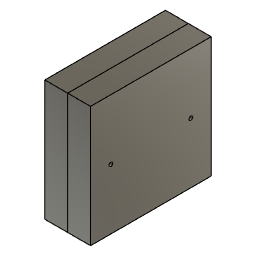
silicone_mold_tyres (Autodesk Fusion 360 design; units mm, degrees)
Autodesk Fusion 360 part; units mm, degrees
note: some values were not read from the file. Set by a fixed rule: which face or edge a step refers to.
sketch "Sketch1" plane through (0, 0, 0) normal (0, 0, 1) x (1, 0, 0)
  circle A0 centre (0, 0) radius 25
  dimension "d1" = 50
  constraint coincident A0.centre origin
  measures "d1" diameter of A0
extrude "Extrude1" add sketch "Sketch1" along normal blind 18 makes body 1
move_body "Move1" bodies 1 to x (0, 0, 1) y (0, 1, 0) z (-1, 0, 0) at (18, 0, 18)
fillet "Fillet1" radius 4 2 edges at (0, -9.0404, -5.3082) (18, -9.0404, -5.3082) on bodies 1
ref_plane "WorkPlane1" through (9, 0, 18) normal (1, 0, 0) x (0, 0, -1)
sketch "Sketch2" plane through (9, 0, 18) normal (1, 0, 0) x (0, 1, 0)
  line L0 (0, 0) -> (-26.2939, 0)
  circle A0 centre (0, 0) radius 26.2939
  circle A1 centre (0, 0) radius 25
  circle A2 centre (0, 0) radius 25
  constraint coincident L0.start A0.centre
  constraint horizontal L0
  constraint coincident L0.end A0
extrude "Extrude2" add sketch "Sketch2" along normal mid plane 9.2 separate body makes body 2
move_face "OffsetFaces1" offset -0.5 1 faces at (7.4667, -26.1632, 15.382) on bodies 2
sketch "Sketch3" plane through (0, 0, 0) normal (0, 1, 0) x (1, 0, 0)
  line L0 (-4.0723, -11.8438) -> (22.6184, -22.2298)
  line L1 (-4.767, -13.6293) -> (21.9237, -24.0153)
  line L2 (21.9237, -24.0153) -> (22.6184, -22.2298)
  line L3 (-4.767, -13.6293) -> (-4.0723, -11.8438)
  line L4 (4.4, 7.7939) -> (4.4, -43.7939)
  line L5 (13.6, -43.7939) -> (13.6, 7.7939)
  circle A0 through (4, 7, 0) (4, -30.5, 21.6506) (4, -30.5, -21.6506)
  line L6 (4, -18) -> (24.1536, -18)
  line L7 (-4.0723, -24.1562) -> (22.6184, -13.7702)
  line L8 (-4.767, -22.3707) -> (-4.0723, -24.1562)
  line L9 (-4.767, -22.3707) -> (21.9237, -11.9847)
  line L10 (21.9237, -11.9847) -> (22.6184, -13.7702)
  dimension "d9" = 1.9159
  constraint perpendicular L0 L2
  constraint perpendicular L0 L3
  constraint perpendicular L4 L6
  constraint symmetric L0.start L6 L7.start
  constraint symmetric L0.end L6 L7.end
  constraint symmetric L1.start L6 L8.start
  constraint symmetric L1.end L6 L9.end
extrude "Extrude3" cut sketch "Sketch3" against normal blind 58 contours L0 L1 L3 L4 | L0 L1 L4 L9 | L0 L6 L9 | L1 L6 L7 | L0 L1 L5 L7 | L0 L1 L2 L5 keep common part bodies 2
pattern_circular "C-Pattern1" count 23 over 360 about axis through (14, 0, 18) along (-1, 0, 0) of bodies 2 makes body 3 at (7.9822, -24.2718, 23.9901) makes body 4 at (7.9822, -21.7556, 30.3164) makes body 5 at (7.9822, -17.6259, 35.7293) makes body 6 at (7.9822, -12.189, 39.8272) makes body 7 at (7.9822, -5.8481, 42.3064) makes body 8 at (7.9822, 0.9265, 42.9828) makes body 9 at (7.9822, 7.6325, 41.8064) makes body 10 at (7.9822, 13.7723, 38.8644) makes body 11 at (7.9822, 18.8908, 34.375) makes body 12 at (7.9822, 22.6081, 28.6711) makes body 13 at (7.9822, 24.6488, 22.1757) makes body 14 at (7.9822, 24.8614, 15.3707) makes body 15 at (7.9822, 23.2301, 8.7607) makes body 16 at (7.9822, 19.8759, 2.8359) makes body 17 at (7.9822, 15.0476, -1.9642) makes body 18 at (7.9822, 9.1034, -5.2837) makes body 19 at (7.9822, 2.4839, -6.8763) makes body 20 at (7.9822, -4.3197, -6.624) makes body 21 at (7.9822, -10.803, -4.5454) makes body 22 at (7.9822, -16.4851, -0.7947) makes body 23 at (7.9822, -20.9445, 4.3499) makes body 24 at (7.9822, -23.8506, 10.5068)
sketch "Sketch4" plane through (0, 0, 0) normal (-1, 0, 0) x (0, -1, 0)
  circle A0 centre (0, 18) radius 21
  circle A1 centre (0, 18) radius 17.4465
  constraint concentric A0 A1
extrude "Extrude4" cut sketch "Sketch4" against normal blind 40 contours A1 bodies 1
sketch "Sketch5" plane through (0, 0, 0) normal (-1, 0, 0) x (0, -1, 0)
  circle A0 centre (0, 18) radius 17.4465
  circle A1 centre (0, 18) radius 21
  line L0 (29, 47) -> (-29, 47)
  line L1 (-29, 47) -> (-29, -11)
  line L2 (-29, -11) -> (29, -11)
  line L3 (29, -11) -> (29, 47)
  line L4 (29, 47) -> (-29, -11) construction
  line L5 (-29, 47) -> (29, -11) construction
  point P0 (0, 18)
  dimension "d16" = 58
  dimension "d17" = 58
  constraint horizontal L0
  constraint perpendicular L0 L1
  constraint parallel L0 L2
  constraint parallel L1 L3
  constraint coincident L4 P0
  constraint coincident L5 P0
  constraint coincident P0 A0.centre
  measures "d16" distance of L1.end L2.end
  measures "d17" distance of L0.end L1.end
extrude "Extrude5" add sketch "Sketch5" against normal blind 20 separate body contours A0 | A1 | L0 L1 L2 L3 makes body 25
extrude "Extrude6" add sketch "Sketch5" along normal blind 2 separate body contours A0 | A1 | L0 L1 L2 L3 makes body 26
combine "Combine1" operation add target body 25 tool bodies 26
combine "Combine2" operation add target body 1 tool bodies 2 9 18 10 11 17 3 7 24 14 12 13 15 16 6 21 4 5 22 23 8 20 19
combine "Combine3" operation add target body 25 tool bodies 1 keep tools
ref_plane "WorkPlane2" through (9, 0, 18) normal (1, 0, 0) x (0, 0, -1)
split "Split1" by plane through (9, 0, 18) normal (1, 0, 0) bodies 25 makes body 27 at (20, 9.6667, 27.6667)
combine "Combine4" operation cut target body 27 tool bodies 1 keep tools
combine "Combine5" operation cut target body 25 tool bodies 1 keep tools
sketch "Sketch6" plane through (9, 0, 0) normal (1, 0, 0) x (0, 1, 0)
  line L0 (-25.775, 18.9864) -> (-24.9805, 18.9864)
  arc A0 (-24.3394, 23.7089) -> (-24.9805, 18.9864) centre (0, 18) ccw
  line L1 (-24.3394, 23.7089) -> (-25.1046, 23.9233)
  arc A1 (-24.5531, 25.9038) -> (-25.1046, 23.9233) centre (0, 18) ccw
  line L2 (-24.5531, 25.9038) -> (-23.7881, 25.6895)
  arc A2 (-21.8966, 30.0639) -> (-23.7881, 25.6895) centre (0, 18) ccw
  line L3 (-21.8966, 30.0639) -> (-22.5755, 30.4768)
  arc A3 (-21.5102, 32.2351) -> (-22.5755, 30.4768) centre (0, 18) ccw
  line L4 (-21.5102, 32.2351) -> (-20.8313, 31.8223)
  arc A4 (-17.8298, 35.5242) -> (-20.8313, 31.8223) centre (0, 18) ccw
  line L5 (-17.8298, 35.5242) -> (-18.3722, 36.1049)
  arc A5 (-16.872, 37.5106) -> (-18.3722, 36.1049) centre (0, 18) ccw
  line L6 (-16.872, 37.5106) -> (-16.3297, 36.9299)
  arc A6 (-12.4407, 39.6848) -> (-16.3297, 36.9299) centre (0, 18) ccw
  line L7 (-12.4407, 39.6848) -> (-12.8062, 40.3903)
  arc A7 (-10.9824, 41.3391) -> (-12.8062, 40.3903) centre (0, 18) ccw
  line L8 (-10.9824, 41.3391) -> (-10.6169, 40.6336)
  arc A8 (-6.1288, 42.2371) -> (-10.6169, 40.6336) centre (0, 18) ccw
  line L9 (-6.1288, 42.2371) -> (-6.2905, 43.0151)
  arc A9 (-4.2783, 43.4366) -> (-6.2905, 43.0151) centre (0, 18) ccw
  line L10 (-4.2783, 43.4366) -> (-4.1167, 42.6587)
  arc A10 (0.6375, 42.9919) -> (-4.1167, 42.6587) centre (0, 18) ccw
  line L11 (0.6375, 42.9919) -> (0.6918, 43.7846)
  arc A11 (2.743, 43.6476) -> (0.6918, 43.7846) centre (0, 18) ccw
  line L12 (2.743, 43.6476) -> (2.6888, 42.855)
  arc A12 (7.3566, 41.8931) -> (2.6888, 42.855) centre (0, 18) ccw
  line L13 (7.3566, 41.8931) -> (7.6227, 42.6418)
  arc A13 (9.561, 41.9565) -> (7.6227, 42.6418) centre (0, 18) ccw
  line L14 (9.561, 41.9565) -> (9.2949, 41.2079)
  arc A14 (13.5301, 39.0223) -> (9.2949, 41.2079) centre (0, 18) ccw
  line L15 (13.5301, 39.0223) -> (13.9883, 39.6715)
  arc A15 (15.6698, 38.4886) -> (13.9883, 39.6715) centre (0, 18) ccw
  line L16 (15.6698, 38.4886) -> (15.2116, 37.8395)
  arc A16 (18.7001, 34.5924) -> (15.2116, 37.8395) centre (0, 18) ccw
  line L17 (18.7001, 34.5924) -> (19.3165, 35.0938)
  arc A17 (20.6165, 33.5012) -> (19.3165, 35.0938) centre (0, 18) ccw
  line L18 (20.6165, 33.5012) -> (20.0002, 32.9998)
  arc A18 (22.4832, 28.9318) -> (20.0002, 32.9998) centre (0, 18) ccw
  line L19 (22.4832, 28.9318) -> (23.212, 29.2484)
  arc A19 (24.0341, 27.3641) -> (23.212, 29.2484) centre (0, 18) ccw
  line L20 (24.0341, 27.3641) -> (23.3054, 27.0476)
  arc A20 (24.5989, 22.4606) -> (23.3054, 27.0476) centre (0, 18) ccw
  line L21 (24.5989, 22.4606) -> (25.3861, 22.5688)
  arc A21 (25.6693, 20.5325) -> (25.3861, 22.5688) centre (0, 18) ccw
  line L22 (25.6693, 20.5325) -> (24.8822, 20.4243)
  arc A22 (24.8901, 15.6585) -> (24.8822, 20.4243) centre (0, 18) ccw
  line L23 (24.8901, 15.6585) -> (25.6773, 15.5503)
  arc A23 (25.4007, 13.5131) -> (25.6773, 15.5503) centre (0, 18) ccw
  line L24 (25.4007, 13.5131) -> (24.6136, 13.6213)
  arc A24 (23.3354, 9.03) -> (24.6136, 13.6213) centre (0, 18) ccw
  line L25 (23.3354, 9.03) -> (24.0642, 8.7134)
  arc A25 (23.2482, 6.8265) -> (24.0642, 8.7134) centre (0, 18) ccw
  line L26 (23.2482, 6.8265) -> (22.5195, 7.143)
  arc A26 (20.05, 3.0668) -> (22.5195, 7.143) centre (0, 18) ccw
  line L27 (20.05, 3.0668) -> (20.6663, 2.5654)
  arc A27 (19.3715, 0.9685) -> (20.6663, 2.5654) centre (0, 18) ccw
  line L28 (19.3715, 0.9685) -> (18.7552, 1.4699)
  arc A28 (15.2775, -1.7888) -> (18.7552, 1.4699) centre (0, 18) ccw
  line L29 (15.2775, -1.7888) -> (15.7358, -2.438)
  arc A29 (14.0581, -3.6262) -> (15.7358, -2.438) centre (0, 18) ccw
  line L30 (14.0581, -3.6262) -> (13.5999, -2.9772)
  arc A30 (9.372, -5.1768) -> (13.5999, -2.9772) centre (0, 18) ccw
  line L31 (9.372, -5.1768) -> (9.6381, -5.9255)
  arc A31 (7.7021, -6.6171) -> (9.6381, -5.9255) centre (0, 18) ccw
  line L32 (7.7021, -6.6171) -> (7.436, -5.8685)
  arc A32 (2.7715, -6.8459) -> (7.436, -5.8685) centre (0, 18) ccw
  line L33 (2.7715, -6.8459) -> (2.8257, -7.6387)
  arc A33 (0.7749, -7.7823) -> (2.8257, -7.6387) centre (0, 18) ccw
  line L34 (0.7749, -7.7823) -> (0.7207, -6.9896)
  arc A34 (-4.0346, -6.6723) -> (0.7207, -6.9896) centre (0, 18) ccw
  line L35 (-4.0346, -6.6723) -> (-4.1963, -7.4503)
  arc A35 (-6.2098, -7.0352) -> (-4.1963, -7.4503) centre (0, 18) ccw
  line L36 (-6.2098, -7.0352) -> (-6.0482, -6.2574)
  arc A36 (-10.5415, -4.6688) -> (-6.0482, -6.2574) centre (0, 18) ccw
  line L37 (-10.5415, -4.6688) -> (-10.9071, -5.3744)
  arc A37 (-12.734, -4.4315) -> (-10.9071, -5.3744) centre (0, 18) ccw
  line L38 (-12.734, -4.4315) -> (-12.3685, -3.726)
  arc A38 (-16.2666, -0.9841) -> (-12.3685, -3.726) centre (0, 18) ccw
  line L39 (-16.2666, -0.9841) -> (-16.809, -1.5649)
  arc A39 (-18.3137, -0.1641) -> (-16.809, -1.5649) centre (0, 18) ccw
  line L40 (-18.3137, -0.1641) -> (-17.7714, 0.4166)
  arc A40 (-20.7853, 4.1085) -> (-17.7714, 0.4166) centre (0, 18) ccw
  line L41 (-20.7853, 4.1085) -> (-21.4642, 3.6957)
  arc A41 (-22.5352, 5.4505) -> (-21.4642, 3.6957) centre (0, 18) ccw
  line L42 (-22.5352, 5.4505) -> (-21.8564, 5.8633)
  arc A42 (-23.7624, 10.2314) -> (-21.8564, 5.8633) centre (0, 18) ccw
  line L43 (-23.7624, 10.2314) -> (-24.5275, 10.0171)
  arc A43 (-25.0853, 11.9958) -> (-24.5275, 10.0171) centre (0, 18) ccw
  line L44 (-25.0853, 11.9958) -> (-24.3203, 12.2101)
  arc A44 (-24.9771, 16.9305) -> (-24.3203, 12.2101) centre (0, 18) ccw
  line L45 (-24.9771, 16.9305) -> (-25.7717, 16.9305)
  arc A45 (-25.775, 18.9864) -> (-25.7717, 16.9305) centre (0, 18) ccw
  line L46 (29, 47) -> (-29, 47)
  line L47 (-29, 47) -> (-29, -11)
  line L48 (-29, -11) -> (29, -11)
  line L49 (29, -11) -> (29, 47)
  circle A46 centre (-24.199, 42.344) radius 1.7482
  line L50 (0, 60.0685) -> (0, 50.7805)
  circle A47 centre (24.199, 42.344) radius 1.7482
  line L51 (29, 18) -> (48.241, 18)
  circle A48 centre (24.199, -6.344) radius 1.7482
  circle A49 centre (-24.199, -6.344) radius 1.7482
  constraint perpendicular L46 L50
  constraint symmetric A46 L50 A47
  constraint midpoint L49 L51.start
  constraint perpendicular L49 L51
  constraint symmetric A46 L51 A49
  constraint symmetric A47 L51 A48
extrude "Extrude7" add sketch "Sketch6" along normal blind 3 contours A46 | A47 | A48 | A49 bodies 25
combine "Combine6" operation cut target body 27 tool bodies 25 keep tools
sketch "Sketch7" plane through (18, 0, 0) normal (-1, 0, 0) x (0, -1, 0)
  circle A0 centre (0, 18) radius 17.4465
  circle A1 centre (0, 18) radius 21
  line L0 (0, 18) -> (0, 25.2147)
  circle A2 centre (19.2233, 18) radius 0.9
  circle A3 centre (-19.2233, 18) radius 0.9
  dimension "d24" = 1.8
  constraint coincident A0.centre A1.centre
  constraint symmetric L0 A2 A3
  measures "d24" diameter of A2
extrude "Extrude8" cut sketch "Sketch7" along normal mid plane 22 contours A2 | A3 bodies 27
draft "Draft1" angle 5 neutral plane through (9, 0, 18) pull (1, 0, 0) 1 faces at (11, 25.9451, 42.2568) on bodies 25
draft "Draft2" angle 5 neutral plane through (9, 0, 18) pull (1, 0, 0) 1 faces at (11, -22.453, 42.2568) on bodies 25
draft "Draft3" angle 5 neutral plane through (9, 0, 18) pull (1, 0, 0) 1 faces at (11, 25.9451, -6.4311) on bodies 25
draft "Draft4" angle 5 neutral plane through (9, 0, 18) pull (1, 0, 0) 1 faces at (11, -22.453, -6.4311) on bodies 25
sketch "Sketch8" plane through (9, 0, 0) normal (1, 0, 0) x (0, 1, 0)
  circle A0 centre (0, 18) radius 17.4465
  circle A1 centre (0, 18) radius 16.2886
  line L0 (0, 18) -> (17.4465, 18)
  line L1 (0, 18) -> (15.2076, 26.5505)
  line L2 (0, 18) -> (-8.5505, 33.2076)
  line L3 (0, 18) -> (0, 35.4465)
  line L4 (0, 18) -> (-15.2076, 9.4495)
  line L5 (0, 18) -> (-17.4465, 18)
  line L6 (0, 18) -> (8.5505, 2.7924)
  line L7 (0, 18) -> (0, 0.5535)
  dimension "d36" = 360
  constraint concentric A0 A1
  constraint coincident A0.centre A1.centre
  constraint coincident A0 L0.end
  constraint horizontal L0
  constraint coincident A0 L1.end
extrude "Extrude9" cut sketch "Sketch8" against normal blind 9 contours A0 A1 L0 L1 | A0 A1 L6 L7 | A0 A1 L2 L3 | A0 A1 L4 L5 bodies 25
extrude "Extrude10" cut sketch "Sketch8" along normal blind 9 contours A0 A1 L0 L1 | A0 A1 L6 L7 | A0 A1 L2 L3 | A0 A1 L4 L5 bodies 27
sketch "Sketch9" plane through (0, 0, 0) normal (-1, 0, 0) x (0, -1, 0)
  circle A0 centre (0, 18) radius 17.4465
  circle A1 centre (0, 18) radius 21
extrude "Extrude11" add sketch "Sketch9" against normal blind 18 separate body contours A0 makes body 28
ref_plane "WorkPlane3" through (9, 0, 18) normal (1, 0, 0) x (0, 1, 0)
sketch "Sketch10" plane through (9, 0, 18) normal (1, 0, 0) x (0, 1, 0)
  circle A0 centre (0, 0) radius 17.4465
  circle A1 centre (0, 0) radius 18.4465
  dimension "d43" = 36.893
  constraint coincident A0.centre A1.centre
  measures "d43" diameter of A1
extrude "Extrude12" add sketch "Sketch10" along normal mid plane 10 bodies 28
sketch "Sketch11" plane through (18, 0, 0) normal (1, 0, 0) x (0, 1, 0)
  circle A0 centre (0, 18) radius 17.4465
  circle A1 centre (0, 18) radius 18.4465
  line L0 (1.2162, 35.4041) -> (1.2859, 36.4016)
  line L1 (0, 18) -> (0, 26.9514)
  line L2 (-1.2162, 35.4041) -> (-1.2859, 36.4016)
  arc A2 (1.2162, 35.4041) -> (-1.2162, 35.4041) centre (0, 18) ccw
  arc A3 (1.2859, 36.4016) -> (-1.2859, 36.4016) centre (0, 18) ccw
  arc A4 (-6.8256, 35.1372) -> (-9.1427, 34.0214) centre (0, 18) ccw
  line L3 (-8.6471, 33.1529) -> (-9.1427, 34.0214)
  arc A5 (-6.4556, 34.2082) -> (-8.6471, 33.1529) centre (0, 18) ccw
  line L4 (-6.4556, 34.2082) -> (-6.8256, 35.1372)
  arc A6 (-13.5852, 30.4786) -> (-15.1887, 28.4679) centre (0, 18) ccw
  line L5 (-14.3653, 27.9004) -> (-15.1887, 28.4679)
  arc A7 (-12.8488, 29.8021) -> (-14.3653, 27.9004) centre (0, 18) ccw
  line L6 (-12.8488, 29.8021) -> (-13.5852, 30.4786)
  arc A8 (-17.6541, 23.3484) -> (-18.2264, 20.8411) centre (0, 18) ccw
  line L7 (-17.2384, 20.6871) -> (-18.2264, 20.8411)
  arc A9 (-16.6971, 23.0585) -> (-17.2384, 20.6871) centre (0, 18) ccw
  line L8 (-16.6971, 23.0585) -> (-17.6541, 23.3484)
  arc A10 (-18.2264, 15.1589) -> (-17.6541, 12.6516) centre (0, 18) ccw
  line L9 (-16.6971, 12.9415) -> (-17.6541, 12.6516)
  arc A11 (-17.2384, 15.3129) -> (-16.6971, 12.9415) centre (0, 18) ccw
  line L10 (-17.2384, 15.3129) -> (-18.2264, 15.1589)
  arc A12 (-15.1887, 7.5321) -> (-13.5852, 5.5214) centre (0, 18) ccw
  line L11 (-12.8488, 6.1979) -> (-13.5852, 5.5214)
  arc A13 (-14.3653, 8.0996) -> (-12.8488, 6.1979) centre (0, 18) ccw
  line L12 (-14.3653, 8.0996) -> (-15.1887, 7.5321)
  arc A14 (-9.1427, 1.9786) -> (-6.8256, 0.8628) centre (0, 18) ccw
  line L13 (-6.4556, 1.7918) -> (-6.8256, 0.8628)
  arc A15 (-8.6471, 2.8471) -> (-6.4556, 1.7918) centre (0, 18) ccw
  line L14 (-8.6471, 2.8471) -> (-9.1427, 1.9786)
  arc A16 (-1.2859, -0.4016) -> (1.2859, -0.4016) centre (0, 18) ccw
  line L15 (1.2162, 0.5959) -> (1.2859, -0.4016)
  arc A17 (-1.2162, 0.5959) -> (1.2162, 0.5959) centre (0, 18) ccw
  line L16 (-1.2162, 0.5959) -> (-1.2859, -0.4016)
  arc A18 (6.8256, 0.8628) -> (9.1427, 1.9786) centre (0, 18) ccw
  line L17 (8.6471, 2.8471) -> (9.1427, 1.9786)
  arc A19 (6.4556, 1.7918) -> (8.6471, 2.8471) centre (0, 18) ccw
  line L18 (6.4556, 1.7918) -> (6.8256, 0.8628)
  arc A20 (13.5852, 5.5214) -> (15.1887, 7.5321) centre (0, 18) ccw
  line L19 (14.3653, 8.0996) -> (15.1887, 7.5321)
  arc A21 (12.8488, 6.1979) -> (14.3653, 8.0996) centre (0, 18) ccw
  line L20 (12.8488, 6.1979) -> (13.5852, 5.5214)
  arc A22 (17.6541, 12.6516) -> (18.2264, 15.1589) centre (0, 18) ccw
  line L21 (17.2384, 15.3129) -> (18.2264, 15.1589)
  arc A23 (16.6971, 12.9415) -> (17.2384, 15.3129) centre (0, 18) ccw
  line L22 (16.6971, 12.9415) -> (17.6541, 12.6516)
  arc A24 (18.2264, 20.8411) -> (17.6541, 23.3484) centre (0, 18) ccw
  line L23 (16.6971, 23.0585) -> (17.6541, 23.3484)
  arc A25 (17.2384, 20.6871) -> (16.6971, 23.0585) centre (0, 18) ccw
  line L24 (17.2384, 20.6871) -> (18.2264, 20.8411)
  arc A26 (15.1887, 28.4679) -> (13.5852, 30.4786) centre (0, 18) ccw
  line L25 (12.8488, 29.8021) -> (13.5852, 30.4786)
  arc A27 (14.3653, 27.9004) -> (12.8488, 29.8021) centre (0, 18) ccw
  line L26 (14.3653, 27.9004) -> (15.1887, 28.4679)
  arc A28 (9.1427, 34.0214) -> (6.8256, 35.1372) centre (0, 18) ccw
  line L27 (6.4556, 34.2082) -> (6.8256, 35.1372)
  arc A29 (8.6471, 33.1529) -> (6.4556, 34.2082) centre (0, 18) ccw
  line L28 (8.6471, 33.1529) -> (9.1427, 34.0214)
  dimension "d47" = 360
  constraint coincident A0.centre A1.centre
  constraint coincident A1 L0.end
  constraint vertical L1
  constraint symmetric L0.end L1 L2.end
  constraint coincident A0 L2.start
  constraint coincident A0 L0.start
extrude "Extrude13" cut sketch "Sketch11" against normal blind 58 contours A0 A1 L21 L24 | A0 A1 L23 L26 | A0 A1 L19 L22 | A0 A1 L25 L28 | A0 A1 L17 L20 | A0 A1 L0 L27 | A0 A1 L15 L18 | A0 A1 L2 L4 | A0 A1 L13 L16 | A0 A1 L3 L6 | A0 A1 L11 L14 | A0 A1 L5 L8 | A0 A1 L9 L12 | A0 A1 L7 L10 bodies 28
sketch "Sketch12" plane through (0, 0, 0) normal (-1, 0, 0) x (0, -1, 0)
  circle A0 centre (0, 18) radius 17.4465
  circle A1 centre (0, 18) radius 1
  dimension "d50" = 2
  constraint concentric A0 A1
  measures "d50" diameter of A1
extrude "Extrude14" cut sketch "Sketch12" against normal blind 9 contours A1 bodies 28
move_face "OffsetFaces2" offset -0.5 1 faces at (3, -0.995, 17.9004) on bodies 28
delete_face "DeleteFace1" 9 faces at (12, 14.3952, 27.857) (15, 14.526, 25.3699) (12, 9.857, 3.6048) (9, 3.2848, 18.723) (12, 0.695, 1.7262) (15, -10.1017, 3.7755) (15, -16.2293, 16.6112) (15, -16.3716, 24.0293) (15, -7.3699, 32.526) on bodies 27
delete_face "DeleteFace2" 9 faces at (9, 3.2848, 18.723) (3, 14.3952, 27.857) (3, -7.3699, 32.526) (6, -16.6215, 23.3016) (3, 14.526, 25.3699) (6, 9.2127, 3.1842) (6, 0.695, 1.7262) (6, -11.8902, 5.2326) (6, -16.2738, 17.305) on bodies 25
sketch "Sketch13" plane through (0, 0, 0) normal (1, 0, 0) x (0, 1, 0)
  circle A0 centre (0, 18) radius 21
  circle A1 centre (0, 18) radius 1.5
  dimension "d54" = 3
  constraint concentric A0 A1
  measures "d54" diameter of A1
extrude "Extrude15" add sketch "Sketch13" along normal blind 8 contours A1 bodies 25
draft "Draft5" angle 3 neutral plane through (0, 0, 18) pull (1, 0, 0) 1 faces at (5.3333, -1.4925, 17.8506) on bodies 25
